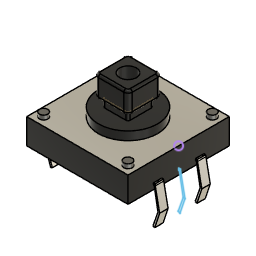
Simple-Embedded-Button v4 (Autodesk Fusion 360 design; units mm, degrees)
Autodesk Fusion 360 part; units mm, degrees
sketch "Sketch1" plane through (0, 0, 0) normal (0, 0, 1) x (1, 0, 0)
  line L0 (6, 6) -> (-6, 6)
  line L1 (-6, 6) -> (-6, -6)
  line L2 (-6, -6) -> (6, -6)
  line L3 (6, -6) -> (6, 6)
  line L4 (6, 6) -> (-6, -6) construction
  line L5 (-6, 6) -> (6, -6) construction
  circle A0 centre (0, 0) radius 3.5
  line L6 (2, 2) -> (-2, 2)
  line L7 (-2, 2) -> (-2, -2)
  line L8 (-2, -2) -> (2, -2)
  line L9 (2, -2) -> (2, 2)
  line L10 (2, 2) -> (-2, -2) construction
  line L11 (-2, 2) -> (2, -2) construction
  circle A1 centre (-5, 5) radius 0.5
  circle A2 centre (5, 5) radius 0.5
  circle A3 centre (-5, -5) radius 0.5
  circle A4 centre (5, -5) radius 0.5
  line L12 (-1.5, -1.5) -> (1.5, -1.5)
  line L13 (1.5, -1.5) -> (1.5, 1.5)
  line L14 (1.5, 1.5) -> (-1.5, 1.5)
  line L15 (-1.5, 1.5) -> (-1.5, -1.5)
  line L16 (-1.5, -1.5) -> (1.5, 1.5) construction
  line L17 (1.5, -1.5) -> (-1.5, 1.5) construction
  circle A5 centre (0, 0) radius 1
  dimension "d1" = 12
  dimension "d2" = 12
  dimension "d3" = 7
  dimension "d4" = 4
  dimension "d5" = 4
  dimension "d14" = 1
  dimension "d15" = 1
  dimension "d16" = 1
  dimension "d17" = 1
  dimension "d21" = 3
  dimension "d22" = 3
  dimension "d34" = 2
  constraint horizontal L0
  constraint perpendicular L0 L1
  constraint parallel L0 L2
  constraint parallel L1 L3
  constraint coincident L4 A0.centre
  constraint coincident L5 A0.centre
  constraint coincident A0.centre A5.centre
  constraint horizontal L6
  constraint perpendicular L6 L7
  constraint parallel L6 L8
  constraint parallel L7 L9
  constraint coincident L10 A0.centre
  constraint coincident L11 A0.centre
  constraint coincident L5 A1.centre
  constraint coincident L4 A2.centre
  constraint coincident L4 A3.centre
  constraint coincident L5 A4.centre
  constraint horizontal L12
  constraint perpendicular L12 L13
  constraint parallel L12 L14
  constraint parallel L13 L15
  constraint coincident L16 A0.centre
  constraint coincident L17 A0.centre
  measures "d1" distance of L1.end L2.end
  measures "d2" distance of L0.end L1.end
  measures "d3" diameter of A0
  measures "d4" distance of L7.end L8.end
  measures "d5" distance of L6.end L7.end
  measures "d14" diameter of A1
  measures "d15" diameter of A2
  measures "d16" diameter of A3
  measures "d17" diameter of A4
  measures "d21" distance of L13.end L14.end
  measures "d22" distance of L12.end L13.end
  measures "d34" diameter of A5
extrude "Extrude1" add sketch "Sketch1" along normal blind 3 contours L0 L1 L2 L3 | A0 | L6 L7 L8 L9 | A1 | A2 | A3 | A4 | L12 L13 L14 L15 | A5 makes body 1
extrude "Extrude2" add sketch "Sketch1" along normal blind 1 from surface at 3 contours A0 | L6 L7 L8 L9 | L12 L13 L14 L15 | A5 bodies 1
extrude "Extrude3" add sketch "Sketch1" along normal blind 1 from surface at 4 contours L12 L13 L14 L15 | A5 bodies 1
extrude "Extrude5" add sketch "Sketch1" along normal blind 2.5 from surface at 5 contours L6 L7 L8 L9 | L12 L13 L14 L15 | A5 bodies 1
fillet "Fillet1" radius 0.5 4 edges at (-2, 2, 6.25) (2, 2, 6.25) (2, -2, 6.25) (-2, -2, 6.25) on bodies 1
fillet "Fillet1" radius 0.25 4 edges at (-2, 0, 7.5) (0, 2, 7.5) (2, 0, 7.5) (0, -2, 7.5) on bodies 1
fillet "Fillet1" radius 0.25 4 edges at (-2, 0, 5) (0, -2, 5) (0, 2, 5) (2, 0, 5) on bodies 1
fillet "Fillet1" radius 0.24 4 edges at (-1.5, 1.5, 4.5) (1.5, 1.5, 4.5) (1.5, -1.5, 4.5) (-1.5, -1.5, 4.5) on bodies 1
extrude "Extrude4" add sketch "Sketch1" along normal blind 0.5 from surface at 3 contours A1 | A2 | A3 | A4 bodies 1
extrude "Extrude6" cut sketch "Sketch1" against normal blind 2 from surface at 7.5 contours A5 bodies 1
sketch "Sketch2" plane through (0, 0, 0) normal (0, 1, 0) x (1, 0, 0)
  line L0 (6, -0.7) -> (6.2, -0.7)
  line L1 (6.2, -0.7) -> (6.7491, 2.0456)
  line L2 (6.7491, 2.0456) -> (6.1601, 3.8273)
  line L3 (6.0889, -0.5337) -> (6.5491, 2.033)
  line L4 (6.5491, 2.033) -> (5.9601, 3.722)
  line L5 (6.1601, 3.8273) -> (5.9601, 3.722)
  line L6 (6.0889, -0.5337) -> (6, -0.5336)
  line L7 (6, -0.5336) -> (6, -0.7)
  point P0 (6, -3)
  dimension "d38" = 2.3
  dimension "d39" = 0.2
  dimension "d40" = 2.8
  dimension "d42" = 0.2
  dimension "d43" = 0.2
  constraint horizontal L0
  measures "d38" distance of L0.start P0
  measures "d39" distance of L0.start L0.end
  measures "d40" distance of L0.end L1.end
  measures "d42" horizontal distance of L1.end L3.end
  measures "d43" horizontal distance of L2.end L4.end
sketch "Sketch3" plane through (6, 0, 0) normal (1, 0, 0) x (0, 1, 0)
  line L0 (-6, 0) -> (6, 0)
  line L1 (6, 0) -> (6, 3)
  line L2 (6, 3) -> (-6, 3)
  line L3 (-6, 3) -> (-6, 0)
  line L4 (-3, 0.6909) -> (-2, 0.6909)
  line L5 (-2, 0.6909) -> (-2, 0.4909)
  line L6 (-2, 0.4909) -> (-3, 0.4909)
  line L7 (-3, 0.4909) -> (-3, 0.6909)
  line L8 (2, 0.6909) -> (3, 0.6909)
  line L9 (3, 0.6909) -> (3, 0.4909)
  line L10 (3, 0.4909) -> (2, 0.4909)
  line L11 (2, 0.4909) -> (2, 0.6909)
  line L12 (0, 3) -> (0, 0)
  dimension "d46" = 1
  dimension "d47" = 0.2
  dimension "d48" = 3
  constraint horizontal L4
  constraint vertical L5
  constraint horizontal L6
  constraint vertical L7
  constraint horizontal L8
  constraint vertical L9
  constraint horizontal L10
  constraint vertical L11
  constraint equal L5 L11
  constraint equal L4 L8
  constraint midpoint L2 L12.start
  constraint coincident L12.end origin
  constraint symmetric L5 L11 L12
  constraint symmetric L4 L8 L12
  measures "d46" distance of L4.start L4.end
  measures "d47" distance of L4.end L5.end
  measures "d48" distance of L3 L7
extrude "Extrude7" add sketch "Sketch3" along normal blind 0.2 contours L4 L5 L6 L7 | L8 L9 L10 L11 bodies 1
extrude "Extrude8" add sketch "Sketch2" along normal up to surface (1 mm away) from surface at -3 separate body makes body 2
extrude "Extrude9" add sketch "Sketch2" along normal up to surface (1 mm away) from surface at 2 separate body makes body 3
ref_plane "WorkPlane1" through (0, 0, 0) normal (1, 0, 0) x (0, 1, 0)
mirror "Mirror1" about plane through (0, 0, 0) normal (1, 0, 0) of bodies 3 2 makes body 4 at (-6.383, -2.6667, -0.2152) makes body 5 at (-6.383, 2.3333, -0.2152)
